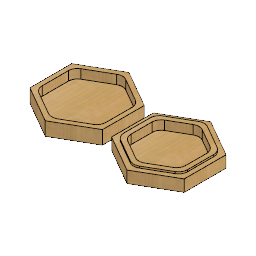
hexbox-v3 (Autodesk Fusion 360 design; units mm, degrees)
Autodesk Fusion 360 part; units mm, degrees
sketch "Sketch1" plane through (0, 0, 0) normal (0, 0, 1) x (1, 0, 0)
  line L0 (50.8, 29.3294) -> (0, 58.6588)
  line L1 (0, 58.6588) -> (-50.8, 29.3294)
  line L2 (-50.8, 29.3294) -> (-50.8, -29.3294)
  line L3 (-50.8, -29.3294) -> (0, -58.6588)
  line L4 (0, -58.6588) -> (50.8, -29.3294)
  line L5 (50.8, -29.3294) -> (50.8, 29.3294)
  line L6 (-6.35, 47.6603) -> (-38.1, 29.3294)
  line L7 (-44.45, 18.3309) -> (-44.45, -18.3309)
  line L8 (-38.1, -29.3294) -> (-6.35, -47.6603)
  line L9 (6.35, -47.6603) -> (38.1, -29.3294)
  line L10 (44.45, -18.3309) -> (44.45, 18.3309)
  line L11 (38.1, 29.3294) -> (6.35, 47.6603)
  line L12 (-6.35, 40.3279) -> (-31.75, 25.6632)
  line L13 (-38.1, 14.6647) -> (-38.1, -14.6647)
  line L14 (-31.75, -25.6632) -> (-6.35, -40.3279)
  line L15 (6.35, -40.3279) -> (31.75, -25.6632)
  line L16 (38.1, -14.6647) -> (38.1, 14.6647)
  line L17 (31.75, 25.6632) -> (6.35, 40.3279)
  arc A0 (-44.45, -18.3309) -> (-38.1, -29.3294) centre (-31.75, -18.3309) ccw
  arc A1 (-38.1, 29.3294) -> (-44.45, 18.3309) centre (-31.75, 18.3309) ccw
  arc A2 (6.35, 47.6603) -> (-6.35, 47.6603) centre (0, 36.6617) ccw
  arc A3 (44.45, 18.3309) -> (38.1, 29.3294) centre (31.75, 18.3309) ccw
  arc A4 (38.1, -29.3294) -> (44.45, -18.3309) centre (31.75, -18.3309) ccw
  arc A5 (-6.35, -47.6603) -> (6.35, -47.6603) centre (0, -36.6617) ccw
  arc A6 (-6.35, -40.3279) -> (6.35, -40.3279) centre (0, -29.3294) ccw
  arc A7 (-38.1, -14.6647) -> (-31.75, -25.6632) centre (-25.4, -14.6647) ccw
  arc A8 (-31.75, 25.6632) -> (-38.1, 14.6647) centre (-25.4, 14.6647) ccw
  arc A9 (6.35, 40.3279) -> (-6.35, 40.3279) centre (0, 29.3294) ccw
  arc A10 (38.1, 14.6647) -> (31.75, 25.6632) centre (25.4, 14.6647) ccw
  arc A11 (31.75, -25.6632) -> (38.1, -14.6647) centre (25.4, -14.6647) ccw
  dimension "d1" = 50.8
  dimension "d16" = 12.7
  measures "d16" radius of A0
extrude "Extrude1" add sketch "Sketch1" along normal blind 6.35 contours L6 L7 L8 L9 L10 L11 A0 A1 A2 A3 A4 A5 | L12 L13 L14 L15 L16 L17 A6 A7 A8 A9 A10 A11 makes body 1
extrude "Extrude2" add sketch "Sketch1" along normal blind 16.51 contours L0 L1 L2 L3 L4 L5 bodies 1
extrude "Extrude3" add sketch "Sketch1" against normal blind 6.35 from surface at 35.56 separate body contours L0 L1 L2 L3 L4 L5 | L6 L7 L8 L9 L10 L11 A0 A1 A2 A3 A4 A5 | L12 L13 L14 L15 L16 L17 A6 A7 A8 A9 A10 A11 makes body 2
extrude "Extrude4" add sketch "Sketch1" against normal blind 12.7 from surface at 29.21 contours L0 L1 L2 L3 L4 L5 bodies 2
extrude "Extrude5" add sketch "Sketch1" along normal blind 19.05 separate body contours L6 L7 L8 L9 L10 L11 A0 A1 A2 A3 A4 A5 makes body 3
combine "Combine1" operation add target body 1 tool bodies 3
move_body "Move1" bodies 2 to x (-1, 0, 0) y (0, 1, 0) z (0, 0, -1) at (-114.3, 0, 35.56)
equation "d3 = 1/4\""
equation "d11 = 0\""
equation "d16 = 1/2\""
